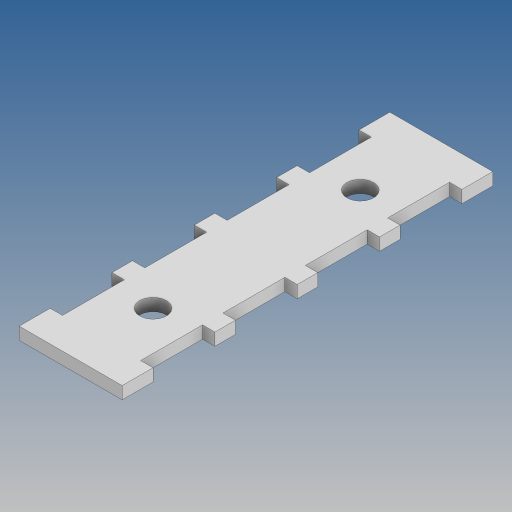
# Autodesk Inventor part: Pieza8
Saved by Autodesk Inventor 2024 (Build 280153000, 153)
## iProperties
Created: 2024-05-31
Part Number: Pieza8
Material: Genérico
Document SubType Name: Modeling
Designer: Pablo
Density: 1 g/cm^3
Appearance: Valor por defecto
Author: Pablo
Autodesk Inventor part; units mm, degrees
ref_plane "YZ Plane" through (0, 0, 0) normal (1, 0, 0) x (0, 1, 0)
ref_plane "XZ Plane" through (0, 0, 0) normal (0, 1, 0) x (-1, 0, 0)
ref_plane "XY Plane" through (0, 0, 0) normal (0, 0, 1) x (1, 0, 0)
sketch "Boceto1" plane through (0, 0, 0) normal (0, 1, 0) x (-1, 0, 0)
  line L0 (0, 2.138) -> (25, 2.138)
  line L1 (25, 2.138) -> (25, -87.862)
  line L2 (25, -87.862) -> (0, -87.862)
  line L3 (0, -87.862) -> (0, 2.138)
  line L4 (0, 2.138) -> (25, -87.862) construction
  line L5 (25, 2.138) -> (0, -87.862) construction
  circle A0 centre (12.5, -17.862) radius 3.25
  circle A1 centre (12.1754, -67.8599) radius 3.25
  line L6 (25, -5.362) -> (22, -5.362)
  line L7 (22, -5.362) -> (22, -20.362)
  line L8 (22, -20.362) -> (25, -20.362)
  line L9 (25, -20.362) -> (25, -5.362)
  line L10 (22, -40.362) -> (25, -40.362)
  line L11 (25, -25.362) -> (22, -25.362)
  line L12 (22, -25.362) -> (22, -40.362)
  line L13 (25, -40.362) -> (25, -25.362)
  line L14 (22, -60.362) -> (25, -60.362)
  line L15 (25, -45.362) -> (22, -45.362)
  line L16 (22, -45.362) -> (22, -60.362)
  line L17 (25, -60.362) -> (25, -45.362)
  line L18 (22, -80.362) -> (25, -80.362)
  line L19 (25, -65.362) -> (22, -65.362)
  line L20 (22, -65.362) -> (22, -80.362)
  line L21 (25, -80.362) -> (25, -65.362)
  line L22 (12.5, 2.138) -> (12.5, -87.862) construction
  line L23 (0, -5.362) -> (3, -5.362)
  line L24 (3, -5.362) -> (3, -20.362)
  line L25 (3, -20.362) -> (0, -20.362)
  line L26 (0, -20.362) -> (0, -5.362)
  line L27 (3, -40.362) -> (0, -40.362)
  line L28 (0, -25.362) -> (3, -25.362)
  line L29 (3, -25.362) -> (3, -40.362)
  line L30 (0, -40.362) -> (0, -25.362)
  line L31 (3, -60.362) -> (0, -60.362)
  line L32 (0, -45.362) -> (3, -45.362)
  line L33 (3, -45.362) -> (3, -60.362)
  line L34 (0, -60.362) -> (0, -45.362)
  line L35 (3, -80.362) -> (0, -80.362)
  line L36 (0, -65.362) -> (3, -65.362)
  line L37 (3, -65.362) -> (3, -80.362)
  line L38 (0, -80.362) -> (0, -65.362)
  point P0 (0, 0)
  point P1 (12.5, -50)
  point P2 (12.5, -42.862)
  point P3 (23.5, -5.362)
  point P4 (23.5, -25.362)
  point P5 (23.5, -45.362)
  point P6 (23.5, -65.362)
  point P7 (1.5, -5.362)
  point P8 (1.5, -25.362)
  point P9 (1.5, -45.362)
  point P10 (1.5, -65.362)
  point P11 (0, -5.362)
  point P12 (12.5, -42.862)
  dimension "d3" = 25
  dimension "d4" = 25
  dimension "d5" = 90
  dimension "d6" = 6.5
  dimension "d7" = 6.5
  dimension "d8" = 3
  dimension "d9" = 15
  dimension "d10" = 7.5
  dimension "d13" = 20
  dimension "d20" = 25
  constraints: 78 end point, 20 symmetric about line, 6 midpoint, 4 parallel, 2 centre point, 2 coincident, 2 horizontal, 2 perpendicular, 1 point on line, 1 vertical, 27 other
  measures "d3" distance of point (12.5, -42.862) point (12.175, -67.86)
  measures "d4" distance of L4.end L3.start
  measures "d5" distance of L5.start L4.end
  measures "d6" diameter of A0
  measures "d7" diameter of A1
  measures "d8" distance of L8.end L7.end
  measures "d9" distance of L7.end L6.end
  measures "d10" distance from line of point (23.5, -5.362) L0
  measures "d13" distance of L7.end L10.start
  measures "d20" distance of point (12.5, -42.862) A0.centre
extrude "Extrusión1" add sketch "Boceto1" along normal blind 3 contours L0 L1 L6 L7 L8 L11 L12 L10 L15 L16 L14 L19 L20 L18 L2 L3 L35 L37 L36 L31 L33 L32 L27 L29 L28 L25 L24 L23
